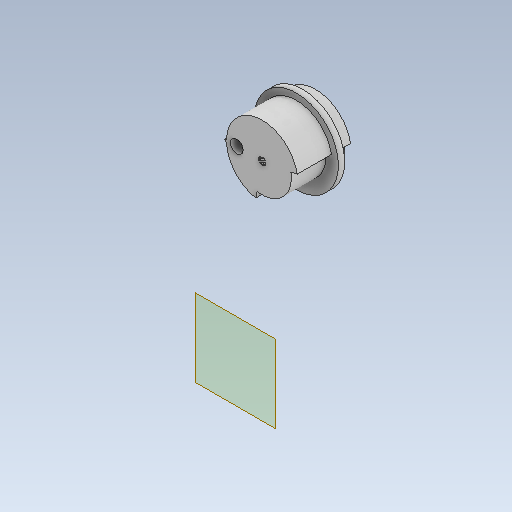
# Autodesk Inventor part: HandleGear2
Saved by Autodesk Inventor 2021 (Build 250183000, 183)
## iProperties
Created: 2021-03-29
Part Number: HandleGear2
Material: Generic
Document SubType Name: Modeling
Designer: ben
Density: 1 g/cm^3
Appearance: Default
Sheet Metal Rule: Default
Author: ben
Autodesk Inventor part; units mm, degrees
ref_plane "YZ Plane" through (0, 0, 0) normal (1, 0, 0) x (0, 1, 0)
ref_plane "XZ Plane" through (0, 0, 0) normal (0, 1, 0) x (-1, 0, 0)
sketch "Sketch1" plane through (0, 0, 0) normal (0, 0, 1) x (1, 0, 0)
  circle A0 centre (52.470893, 183.912819) radius 28
  arc A1 (27.470971, 183.975379) -> (52.408333, 158.912897) centre (52.470893, 183.912819) ccw
  arc A2 (52.408333, 158.912897) -> (52.433357, 168.912866) centre (52.420845, 163.912882) ccw
  arc A3 (37.47094, 183.950355) -> (52.433357, 168.912866) centre (52.470893, 183.912819) ccw
  arc A4 (37.47094, 183.950355) -> (27.470971, 183.975379) centre (32.470955, 183.962867) ccw
  arc A5 (48.476985, 161.262241) -> (75.121471, 187.906727) centre (52.470893, 183.912819) ccw
  line L0 (52.470893, 183.912819) -> (48.476985, 161.262241) construction
  line L1 (52.470893, 183.912819) -> (75.470893, 183.912819) construction
  line L2 (52.470893, 183.912819) -> (75.121471, 187.906727) construction
  line L3 (48.476985, 161.262241) -> (47.608744, 156.338202)
  line L4 (75.121471, 187.906727) -> (80.04551, 188.774968)
  line L5 (55.397568, 184.639605) -> (55.362987, 184.64631)
  line L6 (55.362987, 184.64631) -> (50.081361, 182.12585)
  line L7 (50.081361, 182.12585) -> (50.064822, 182.09475)
  arc A6 (49.616095, 183.035057) -> (50.064822, 182.09475) centre (52.506831, 183.837331) ccw
  line L8 (49.616095, 183.035057) -> (49.650676, 183.028352)
  line L9 (49.650676, 183.028352) -> (54.932302, 185.548812)
  line L10 (54.932302, 185.548812) -> (54.948841, 185.579912)
  arc A7 (55.397568, 184.639605) -> (54.948841, 185.579912) centre (52.506831, 183.837331) ccw
  line L11 (49.516034, 184.07213) -> (50.267232, 183.621245)
  line L12 (50.267232, 183.621245) -> (49.616095, 183.035057)
  arc A8 (49.516034, 184.07213) -> (49.616095, 183.035057) centre (52.506831, 183.837331) ccw
  line L13 (49.776707, 185.080883) -> (50.32839, 184.400265)
  line L14 (50.32839, 184.400265) -> (49.516034, 184.07213)
  arc A9 (49.776707, 185.080883) -> (49.516034, 184.07213) centre (52.506831, 183.837331) ccw
  line L15 (50.366674, 185.939645) -> (50.652301, 185.111387)
  line L16 (50.652301, 185.111387) -> (49.776707, 185.080883)
  arc A10 (50.366674, 185.939645) -> (49.776707, 185.080883) centre (52.506831, 183.837331) ccw
  line L17 (50.366674, 185.939645) -> (50.652301, 185.111387)
  line L18 (50.652301, 185.111387) -> (49.776707, 185.080883)
  arc A11 (50.366674, 185.939645) -> (49.776707, 185.080883) centre (52.506831, 183.837331) ccw
  line L19 (51.199896, 185.668839) -> (50.366674, 185.939645)
  arc A12 (51.214775, 186.544837) -> (50.366674, 185.939645) centre (52.506831, 183.837331) ccw
  line L20 (51.214775, 186.544837) -> (51.199896, 185.668839)
  line L21 (51.905126, 186.005384) -> (51.214775, 186.544837)
  arc A13 (52.218717, 186.823464) -> (51.214775, 186.544837) centre (52.506831, 183.837331) ccw
  line L22 (52.218717, 186.823464) -> (51.905126, 186.005384)
  line L23 (52.682931, 186.080429) -> (52.218717, 186.823464)
  arc A14 (53.25741, 186.741919) -> (52.218717, 186.823464) centre (52.506831, 183.837331) ccw
  line L24 (53.25741, 186.741919) -> (52.682931, 186.080429)
  line L25 (53.439495, 185.884924) -> (53.25741, 186.741919)
  arc A15 (54.205572, 186.310038) -> (53.25741, 186.741919) centre (52.506831, 183.837331) ccw
  line L26 (54.205572, 186.310038) -> (53.439495, 185.884924)
  line L27 (54.948841, 185.579912) -> (54.083567, 185.44245)
  line L28 (54.083567, 185.44245) -> (54.205572, 186.310038)
  arc A16 (54.948841, 185.579912) -> (54.205572, 186.310038) centre (52.506831, 183.837331) ccw
  line L29 (55.497629, 183.602532) -> (54.746431, 184.053417)
  line L30 (54.746431, 184.053417) -> (55.397568, 184.639605)
  arc A17 (55.497629, 183.602532) -> (55.397568, 184.639605) centre (52.506831, 183.837331) ccw
  line L31 (54.685272, 183.274397) -> (55.497629, 183.602532)
  arc A18 (55.236956, 182.593779) -> (55.497629, 183.602532) centre (52.506831, 183.837331) ccw
  line L32 (55.236956, 182.593779) -> (54.685272, 183.274397)
  line L33 (54.361362, 182.563276) -> (55.236956, 182.593779)
  arc A19 (54.646989, 181.735017) -> (55.236956, 182.593779) centre (52.506831, 183.837331) ccw
  line L34 (54.646989, 181.735017) -> (54.361362, 182.563276)
  line L35 (53.813767, 182.005824) -> (54.646989, 181.735017)
  arc A20 (53.798888, 181.129825) -> (54.646989, 181.735017) centre (52.506831, 183.837331) ccw
  line L36 (53.798888, 181.129825) -> (53.813767, 182.005824)
  line L37 (53.108537, 181.669279) -> (53.798888, 181.129825)
  arc A21 (52.794946, 180.851198) -> (53.798888, 181.129825) centre (52.506831, 183.837331) ccw
  line L38 (52.794946, 180.851198) -> (53.108537, 181.669279)
  line L39 (52.330732, 181.594233) -> (52.794946, 180.851198)
  arc A22 (51.756253, 180.932743) -> (52.794946, 180.851198) centre (52.506831, 183.837331) ccw
  line L40 (51.756253, 180.932743) -> (52.330732, 181.594233)
  line L41 (50.808091, 181.364624) -> (51.574167, 181.789738)
  line L42 (51.574167, 181.789738) -> (51.756253, 180.932743)
  arc A23 (50.808091, 181.364624) -> (51.756253, 180.932743) centre (52.506831, 183.837331) ccw
  line L43 (50.064822, 182.09475) -> (50.930096, 182.232213)
  line L44 (50.930096, 182.232213) -> (50.808091, 181.364624)
  arc A24 (50.064822, 182.09475) -> (50.808091, 181.364624) centre (52.506831, 183.837331) ccw
  line L45 (52.506831, 183.837331) -> (24.470995, 183.837331)
  line L46 (22.470995, 183.837331) -> (25.470995, 185.569382)
  line L47 (25.470995, 185.569382) -> (25.470995, 182.10528)
  line L48 (25.470995, 182.10528) -> (22.470995, 183.837331)
  point P0 (0, 0)
  point P1 (24.498637, 182.666672)
  point P2 (24.492173, 185.004259)
  point P3 (10.335246, 8.610376)
  point P4 (51.352392, 183.840433)
  point P5 (50.978828, 182.554133)
  point P6 (-2.300923, 5.12645)
  point P7 (2.854932, 6.911009)
  point P8 (2.854932, 6.911009)
  point P9 (2.028345, 7.54527)
  point P10 (28.297094, 96.837198)
  point P11 (52.600715, 184.436149)
  point P12 (52.235506, 183.153836)
  point P13 (28.297094, 96.837198)
  point P14 (28.409967, 96.755736)
  point P15 (-2.300923, 5.12645)
  point P16 (12.438269, 8.400002)
  point P17 (2.028345, 7.54527)
  point P18 (28.297094, 96.837198)
  point P19 (0.93118, 4.37353)
  point P20 (0.246619, 4.700102)
  point P21 (1.963625, 4.988962)
  point P22 (1.666846, 4.939033)
  point P23 (2.791311, 2.901621)
  point P24 (1.820575, 5.057204)
  point P25 (2.804471, 2.914618)
  point P26 (1.981568, 7.750306)
  point P27 (1.981568, 7.750306)
  point P28 (0.977589, 8.028802)
  point P29 (0.977589, 8.028802)
  point P30 (-0.061093, 7.947121)
  point P31 (-0.061093, 7.947121)
  point P32 (-1.009199, 7.515116)
  point P33 (-1.009199, 7.515116)
  point P34 (-1.724294, 3.261666)
  point P35 (3.618534, 5.267374)
  point P36 (3.640244, 5.015096)
  point P37 (0.02326, 4.832214)
  point P38 (50.037001, 184.759756)
  point P39 (24.970928, 96.884707)
  point P40 (7.748731, 6.162094)
  point P41 (8.009404, 7.170847)
  point P42 (27.35203, 97.268277)
  point P43 (-2.300923, 5.12645)
  point P44 (0.48077, 4.850931)
  point P45 (2.916778, 3.426296)
  point P46 (7.848792, 5.125021)
  point P47 (50.318929, 183.347251)
  point P48 (52.408333, 158.912897)
  point P49 (52.433357, 168.912866)
  point P50 (9.937135, 8.817998)
  dimension "d8" = 23
  dimension "d9" = 100
  dimension "d10" = 110
  dimension "d11" = 4.92404
  dimension "d12" = 4.92404
  dimension "d18" = 3
  constraints: 18 end point, 5 point on circle, 2 horizontal, 1 centre point, 1 coincident, 1 equal length, 1 point on line, 7 other
  measures "d8" radius of A5
  measures "d9" angle of L0 L1
  measures "d10" angle of L0 L2
  measures "d11" horizontal distance of L2.end L4.end
  measures "d12" vertical distance of L0.end L3.end
  measures "d18" horizontal distance of L46.start L46.end
ref_plane "Work Plane1" through (-27.427, -23.110149, -9.628472) normal (0, 0, 1) x (0.9999965, 0.0026331, 0)
sketch "Sketch1 outline for Extrusion3" plane through (0, 0, 0) normal (0, 0, 1) x (1, 0, 0)
  line L0 (47.608744, 156.338202) -> (48.476985, 161.262241)
  arc A0 (48.476985, 161.262241) -> (75.121471, 187.906727) centre (52.470893, 183.912819) ccw
  line L1 (75.121471, 187.906727) -> (80.04551, 188.774968)
  arc A1 (80.04551, 188.774968) -> (24.492173, 185.004259) centre (52.470893, 183.912819) ccw
  line L2 (24.492173, 185.004259) -> (22.470995, 183.837331)
  line L3 (22.470995, 183.837331) -> (24.498637, 182.666672)
  arc A2 (24.498637, 182.666672) -> (47.608744, 156.338202) centre (52.470893, 183.912819) ccw
extrude "Extrusion3" add sketch "Sketch1 outline for Extrusion3" along normal blind -35
sketch "Sketch6" plane through (0, 0, 0) normal (0, 0, 1) x (-1, 0, 0)
  line L0 (-13, 18) -> (15, 18)
  line L1 (15, 18) -> (15, -27)
  line L2 (15, -27) -> (-13, -27)
  line L3 (-13, -27) -> (-13, 18)
  line L4 (-25.470995, -182.10528) -> (-22.470995, -183.837331)
  line L5 (-22.470995, -183.837331) -> (-25.470995, -185.569382)
  arc A0 (-80.04551, -188.774968) -> (-24.492173, -185.004259) centre (-52.470893, -183.912819) ccw
  arc A1 (-24.498637, -182.666672) -> (-47.608744, -156.338202) centre (-52.470893, -183.912819) ccw
  line L6 (-75.121471, -187.906727) -> (-80.04551, -188.774968)
  arc A2 (-75.121471, -187.906727) -> (-48.476985, -161.262241) centre (-52.470893, -183.912819) ccw
  line L7 (-47.608744, -156.338202) -> (-48.476985, -161.262241)
  line L8 (-49.776707, -185.080883) -> (-50.32839, -184.400265)
  line L9 (-50.32839, -184.400265) -> (-49.516034, -184.07213)
  arc A3 (-49.776707, -185.080883) -> (-49.516034, -184.07213) centre (-52.506831, -183.837331) ccw
  line L10 (-50.366674, -185.939645) -> (-50.652301, -185.111387)
  line L11 (-50.652301, -185.111387) -> (-49.776707, -185.080883)
  arc A4 (-50.366674, -185.939645) -> (-49.776707, -185.080883) centre (-52.506831, -183.837331) ccw
  line L12 (-51.199896, -185.668839) -> (-50.366674, -185.939645)
  arc A5 (-51.214775, -186.544837) -> (-50.366674, -185.939645) centre (-52.506831, -183.837331) ccw
  line L13 (-51.214775, -186.544837) -> (-51.199896, -185.668839)
  line L14 (-51.905126, -186.005384) -> (-51.214775, -186.544837)
  arc A6 (-52.218717, -186.823464) -> (-51.214775, -186.544837) centre (-52.506831, -183.837331) ccw
  line L15 (-52.218717, -186.823464) -> (-51.905126, -186.005384)
  line L16 (-52.682931, -186.080429) -> (-52.218717, -186.823464)
  arc A7 (-53.25741, -186.741919) -> (-52.218717, -186.823464) centre (-52.506831, -183.837331) ccw
  line L17 (-53.25741, -186.741919) -> (-52.682931, -186.080429)
  line L18 (-53.439495, -185.884924) -> (-53.25741, -186.741919)
  arc A8 (-54.205572, -186.310038) -> (-53.25741, -186.741919) centre (-52.506831, -183.837331) ccw
  line L19 (-54.205572, -186.310038) -> (-53.439495, -185.884924)
  line L20 (-54.948841, -185.579912) -> (-54.083567, -185.44245)
  line L21 (-54.083567, -185.44245) -> (-54.205572, -186.310038)
  arc A9 (-54.948841, -185.579912) -> (-54.205572, -186.310038) centre (-52.506831, -183.837331) ccw
  line L22 (-54.385616, -185.287927) -> (-50.197361, -183.289238)
  line L23 (-54.932302, -185.548812) -> (-54.385616, -185.287927)
  line L24 (-50.197361, -183.289238) -> (-49.650676, -183.028352)
  line L25 (-50.081361, -182.12585) -> (-50.628047, -182.386736)
  line L26 (-80.599892, -119.580705) -> (-84.788147, -121.579394)
  line L27 (-54.816302, -184.385425) -> (-55.362987, -184.64631)
  line L28 (-55.497629, -183.602532) -> (-54.746431, -184.053417)
  line L29 (-54.746431, -184.053417) -> (-55.397568, -184.639605)
  arc A10 (-55.497629, -183.602532) -> (-55.397568, -184.639605) centre (-52.506831, -183.837331) ccw
  line L30 (-54.685272, -183.274397) -> (-55.497629, -183.602532)
  arc A11 (-55.236956, -182.593779) -> (-55.497629, -183.602532) centre (-52.506831, -183.837331) ccw
  line L31 (-55.236956, -182.593779) -> (-54.685272, -183.274397)
  line L32 (-54.361362, -182.563276) -> (-55.236956, -182.593779)
  arc A12 (-54.646989, -181.735017) -> (-55.236956, -182.593779) centre (-52.506831, -183.837331) ccw
  line L33 (-54.646989, -181.735017) -> (-54.361362, -182.563276)
  line L34 (-53.813767, -182.005824) -> (-54.646989, -181.735017)
  arc A13 (-53.798888, -181.129825) -> (-54.646989, -181.735017) centre (-52.506831, -183.837331) ccw
  line L35 (-53.798888, -181.129825) -> (-53.813767, -182.005824)
  line L36 (-53.108537, -181.669279) -> (-53.798888, -181.129825)
  arc A14 (-52.794946, -180.851198) -> (-53.798888, -181.129825) centre (-52.506831, -183.837331) ccw
  line L37 (-52.794946, -180.851198) -> (-53.108537, -181.669279)
  line L38 (-52.330732, -181.594233) -> (-52.794946, -180.851198)
  arc A15 (-51.756253, -180.932743) -> (-52.794946, -180.851198) centre (-52.506831, -183.837331) ccw
  line L39 (-51.756253, -180.932743) -> (-52.330732, -181.594233)
  line L40 (-50.808091, -181.364624) -> (-51.574167, -181.789738)
  line L41 (-51.574167, -181.789738) -> (-51.756253, -180.932743)
  arc A16 (-50.808091, -181.364624) -> (-51.756253, -180.932743) centre (-52.506831, -183.837331) ccw
  line L42 (-50.064822, -182.09475) -> (-50.930096, -182.232213)
  line L43 (-50.930096, -182.232213) -> (-50.808091, -181.364624)
  arc A17 (-50.064822, -182.09475) -> (-50.808091, -181.364624) centre (-52.506831, -183.837331) ccw
  line L44 (-49.516034, -184.07213) -> (-50.267232, -183.621245)
  line L45 (-50.267232, -183.621245) -> (-49.616095, -183.035057)
  arc A18 (-49.516034, -184.07213) -> (-49.616095, -183.035057) centre (-52.506831, -183.837331) ccw
  line L46 (-14.334062, -0.883373) -> (-14.299481, -0.890078)
  line L47 (-50.064822, -182.09475) -> (-50.081361, -182.12585)
  line L48 (-88.740755, -167.608831) -> (-88.724215, -167.577731)
  line L49 (-20.046373, -2.501331) -> (-20.080954, -2.494626)
  circle A19 centre (-52.470893, -183.912819) radius 23
  point P0 (0, 0)
  point P1 (-25.470995, -185.569382)
  point P2 (1.409842, -93.193831)
  point P3 (1.416305, -95.531419)
  point P4 (15, -17.107983)
  point P5 (-13, -24.372672)
  point P6 (-6.471252, 18)
  point P7 (-80.04551, -188.774968)
  point P8 (-37.894654, -160.006057)
  point P9 (-47.608744, -156.338202)
  point P10 (-24.492173, -185.004259)
  point P11 (-47.608744, -156.338202)
  point P12 (1.798755, -5.482521)
  point P13 (-24.352293, -95.624907)
  point P14 (1.585428, -5.574084)
  point P15 (1.681242, -5.376758)
  point P16 (1.705701, -5.231027)
  point P17 (-24.618882, -95.634194)
  point P18 (-25.093052, -96.260469)
  point P19 (-50.130168, -185.093197)
  point P20 (-3.098801, -6.511985)
  point P21 (2.154323, -4.088379)
  point P22 (2.165212, -4.121471)
  point P23 (-2.338391, -3.702217)
  point P24 (-24.109723, -94.802131)
  point P25 (-23.983412, -94.373693)
  point P26 (-23.757382, -93.607019)
  point P27 (-1.514776, -5.83932)
  point P28 (2.30918, -4.966945)
  point P29 (-2.176676, -6.155187)
  point P30 (-48.476985, -161.262241)
  dimension "d27" = 28
  dimension "d28" = 45
  constraints: 8 end point, 2 parallel, 1 centre point, 1 coincident, 1 concentric, 1 horizontal, 1 perpendicular, 2 other
  measures "d27" distance of L1.end L2.end
  measures "d28" distance of L0.end L1.end
sketch "Sketch6 outline for Extrusion6" plane through (0, 0, 0) normal (0, 0, 1) x (-1, 0, 0)
  arc A0 (-48.476985, -161.262241) -> (-75.121471, -187.906727) centre (-52.470893, -183.912819) ccw
  line L0 (-75.121471, -187.906727) -> (-80.04551, -188.774968)
  arc A1 (-80.04551, -188.774968) -> (-24.492173, -185.004259) centre (-52.470893, -183.912819) ccw
  line L1 (-24.492173, -185.004259) -> (-22.470995, -183.837331)
  line L2 (-22.470995, -183.837331) -> (-24.498637, -182.666672)
  arc A2 (-24.498637, -182.666672) -> (-47.608744, -156.338202) centre (-52.470893, -183.912819) ccw
  line L3 (-47.608744, -156.338202) -> (-48.476985, -161.262241)
  line L4 (-54.948841, -185.579912) -> (-54.932302, -185.548812)
  line L5 (-54.932302, -185.548812) -> (-49.650676, -183.028352)
  line L6 (-49.650676, -183.028352) -> (-49.616095, -183.035057)
  line L7 (-49.616095, -183.035057) -> (-50.267232, -183.621245)
  line L8 (-50.267232, -183.621245) -> (-49.516034, -184.07213)
  line L9 (-49.516034, -184.07213) -> (-50.32839, -184.400265)
  line L10 (-50.32839, -184.400265) -> (-49.776707, -185.080883)
  line L11 (-49.776707, -185.080883) -> (-50.652301, -185.111387)
  line L12 (-50.652301, -185.111387) -> (-50.366674, -185.939645)
  line L13 (-50.366674, -185.939645) -> (-51.199896, -185.668839)
  line L14 (-51.199896, -185.668839) -> (-51.214775, -186.544837)
  line L15 (-51.214775, -186.544837) -> (-51.905126, -186.005384)
  line L16 (-51.905126, -186.005384) -> (-52.218717, -186.823464)
  line L17 (-52.218717, -186.823464) -> (-52.682931, -186.080429)
  line L18 (-52.682931, -186.080429) -> (-53.25741, -186.741919)
  line L19 (-53.25741, -186.741919) -> (-53.439495, -185.884924)
  line L20 (-53.439495, -185.884924) -> (-54.205572, -186.310038)
  line L21 (-54.205572, -186.310038) -> (-54.083567, -185.44245)
  line L22 (-54.083567, -185.44245) -> (-54.948841, -185.579912)
  line L23 (-51.756253, -180.932743) -> (-51.574167, -181.789738)
  line L24 (-51.574167, -181.789738) -> (-50.808091, -181.364624)
  line L25 (-50.808091, -181.364624) -> (-50.930096, -182.232213)
  line L26 (-50.930096, -182.232213) -> (-50.064822, -182.09475)
  line L27 (-50.064822, -182.09475) -> (-50.081361, -182.12585)
  line L28 (-50.081361, -182.12585) -> (-55.362987, -184.64631)
  line L29 (-55.362987, -184.64631) -> (-55.397568, -184.639605)
  line L30 (-55.397568, -184.639605) -> (-54.746431, -184.053417)
  line L31 (-54.746431, -184.053417) -> (-55.497629, -183.602532)
  line L32 (-55.497629, -183.602532) -> (-54.685272, -183.274397)
  line L33 (-54.685272, -183.274397) -> (-55.236956, -182.593779)
  line L34 (-55.236956, -182.593779) -> (-54.361362, -182.563276)
  line L35 (-54.361362, -182.563276) -> (-54.646989, -181.735017)
  line L36 (-54.646989, -181.735017) -> (-53.813767, -182.005824)
  line L37 (-53.813767, -182.005824) -> (-53.798888, -181.129825)
  line L38 (-53.798888, -181.129825) -> (-53.108537, -181.669279)
  line L39 (-53.108537, -181.669279) -> (-52.794946, -180.851198)
  line L40 (-52.794946, -180.851198) -> (-52.330732, -181.594233)
  line L41 (-52.330732, -181.594233) -> (-51.756253, -180.932743)
extrude "Extrusion6" add sketch "Sketch6 outline for Extrusion6" along normal blind 7
ref_plane "Work Plane2" through (0, 0, -25) normal (0, 0, -1) x (1, 0, 0)
sketch "Sketch9" plane through (0, 0, -25) normal (0, 0, -1) x (1, 0, 0)
  arc A0 (79.283605, -175.845697) -> (32.519992, -203.558724) centre (52.470893, -183.912819) ccw
  arc A1 (24.492173, -185.004259) -> (80.04551, -188.774968) centre (52.470893, -183.912819) ccw
  arc A2 (32.519992, -203.558724) -> (79.283605, -175.845697) centre (52.470893, -183.912819) ccw
  arc A3 (60.838676, -151.99135) -> (54.152764, -216.869932) centre (52.470893, -183.912819) ccw
  arc A4 (54.152764, -216.869932) -> (60.838676, -151.99135) centre (52.470893, -183.912819) ccw
  point P0 (0, 0)
  point P1 (-1.409842, -93.193831)
  point P2 (47.608744, -156.338202)
  dimension "d34" = 5
  constraints: 4 point on circle, 2 centre point, 2 other
  measures "d34" radial gap between concentric circles of A2 A4
extrude "Extrusion8" add sketch "Sketch9" against normal blind 5 contours A2 A1 A0 | A4 A3
sketch "Sketch10" plane through (0, 0, -35) normal (0, 0, -1) x (-1, 0, 0)
  circle A0 centre (-52.470893, 183.912819) radius 33
  line L0 (-45.003618, 195.083493) -> (-46.530443, 171.860632)
  line L1 (-46.530443, 171.860632) -> (-65.878618, 184.794332)
  line L2 (-65.878618, 184.794332) -> (-45.003618, 195.083493)
  point P0 (0, 0)
  point P1 (-33.649506, 4.426415)
  point P2 (-18.014678, 33.031434)
  dimension "d37" = 20.875
  constraints: 6 end point, 1 coincident, 8 other
  measures "d37" horizontal distance of L1.end L0.start
extrude "Extrusion9" cut sketch "Sketch10" against normal blind 15 contours L0 L1 L2
sketch "Sketch14" plane through (52.470893, 183.912819, 7) normal (0, 0, 1) x (0.7071068, 0.7071068, 0)
  arc A0 (-10.580026, 10.633111) -> (-17.633377, 17.721851) centre (-14.106702, 14.177481) ccw
  circle A1 centre (-14.106702, 14.177481) radius 5
  point P0 (-17.633377, 17.721851)
  point P1 (-9.106702, 14.177481)
  dimension "d44" = 10
  constraints: 1 centre point, 1 coincident
  measures "d44" diameter of A1
extrude "Extrusion11" cut sketch "Sketch14" against normal blind 25
sketch "Sketch15" plane through (0, 0, -35) normal (0, 0, -1) x (-1, 0, 0)
  line L0 (-45.003618, 195.083493) -> (-46.530443, 171.860632)
  line L1 (-46.530443, 171.860632) -> (-65.878618, 184.794332)
  line L2 (-65.878618, 184.794332) -> (-45.003618, 195.083493)
  arc A0 (-47.608744, 156.338202) -> (-24.498637, 182.666672) centre (-52.470893, 183.912819) ccw
  line L3 (-24.498637, 182.666672) -> (-22.470995, 183.837331)
  line L4 (-22.470995, 183.837331) -> (-24.492173, 185.004259)
  arc A1 (-24.492173, 185.004259) -> (-80.04551, 188.774968) centre (-52.470893, 183.912819) ccw
  line L5 (-80.04551, 188.774968) -> (-75.121471, 187.906727)
  arc A2 (-75.121471, 187.906727) -> (-48.476985, 161.262241) centre (-52.470893, 183.912819) ccw
  line L6 (-48.476985, 161.262241) -> (-47.608744, 156.338202)
  circle A3 centre (-52.470893, 183.912819) radius 28
  point P0 (0, 0)
  point P1 (-24.498637, 182.666672)
  constraints: 1 centre point, 1 coincident
extrude "Extrusion12" cut sketch "Sketch15" against normal up to surface (10 mm away) contours A3 L4 L3
equation "\"BendRadius\" = Thickness"
equation "\"BendReliefWidth\" = Thickness"
equation "\"BendReliefDepth\" = 0.5 * Thickness"
equation "\"CornerReliefSize\" = 4 * Thickness"
equation "\"MinimumRemnant\" = 2 * Thickness"
equation "\"TransitionRadius\" = BendRadius"
equation "\"JacobiRadiusSize\" = Thickness"
equation "\"GapSize\" = Thickness"
equation "\"Thickness\" = 0.5"
body "Solid3"
